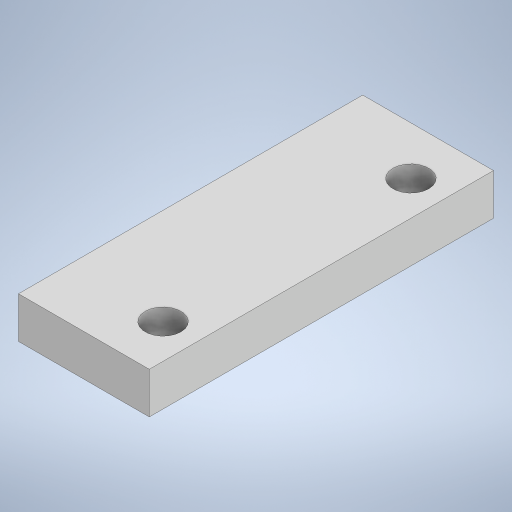
# Autodesk Inventor part: Fuhrungschiene(n)
Saved by Autodesk Inventor 2023 (Build 270158000, 158)
## iProperties
Created: 2023-05-10
Part Number: Fuhrungschiene(n)
Material: Generic
Document SubType Name: Modeling
Designer: dell
Density: 1 g/cm^3
Appearance: Default
Author: dell
Autodesk Inventor part; units mm, degrees
ref_plane "YZ Plane" through (0, 0, 0) normal (1, 0, 0) x (0, 1, 0)
ref_plane "XZ Plane" through (0, 0, 0) normal (0, 1, 0) x (-1, 0, 0)
ref_plane "XY Plane" through (0, 0, 0) normal (0, 0, 1) x (1, 0, 0)
sketch "Sketch1" plane through (0, 0, 0) normal (0, 1, 0) x (-1, 0, 0)
  line L0 (9.5, 25) -> (-9.5, 25)
  line L1 (-9.5, 25) -> (-9.5, -25)
  line L2 (-9.5, -25) -> (9.5, -25)
  line L3 (9.5, -25) -> (9.5, 25)
  line L4 (9.5, 25) -> (-9.5, -25) construction
  line L5 (-9.5, 25) -> (9.5, -25) construction
  circle A0 centre (-4.5, -18) radius 2.6
  circle A1 centre (-4.5, 18) radius 2.6
  point P0 (0, 0)
  dimension "d0" = 50
  dimension "d1" = 19
  dimension "d2" = 5.2
  dimension "d3" = 5.2
  dimension "d4" = 36
  dimension "d5" = 5
  dimension "d6" = 18
  constraints: 12 end point, 2 centre point, 2 midpoint, 2 parallel, 1 horizontal, 1 perpendicular
  measures "d0" distance of L2.end L0.start
  measures "d1" distance of L1.end L2.end
  measures "d2" diameter of A0
  measures "d3" diameter of A1
  measures "d4" distance of A1.centre A0.centre
  measures "d5" distance from line of L1 A1.centre
  measures "d6" vertical distance of point (0, 0) A0.centre
extrude "Extrusion1" add sketch "Sketch1" along normal blind 6
body "Solid1"
